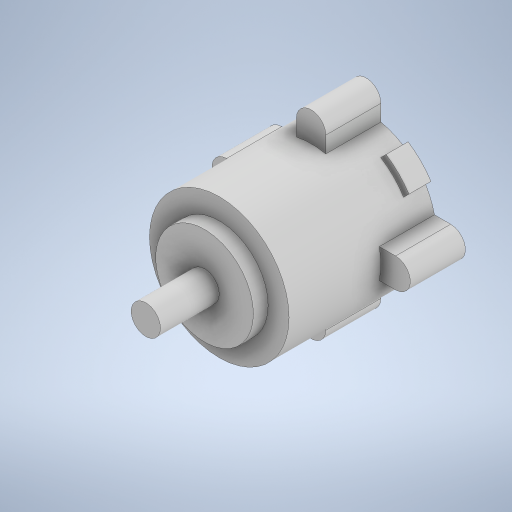
# Autodesk Inventor part: Solenoid Valve
Saved by Autodesk Inventor 2023 (Build 270158000, 158)
## iProperties
Created: 2024-03-20
Part Number: Solenoid Valve
Material: Generic
Document SubType Name: Modeling
Designer: Pobe Tran
Density: 1 g/cm^3
Appearance: Default
Author: Pobe Tran
Autodesk Inventor part; units mm, degrees
ref_plane "YZ Plane" through (0, 0, 0) normal (1, 0, 0) x (0, 1, 0)
ref_plane "XZ Plane" through (0, 0, 0) normal (0, 1, 0) x (-1, 0, 0)
ref_plane "XY Plane" through (0, 0, 0) normal (0, 0, 1) x (1, 0, 0)
sketch "Sketch1" plane through (0, 0, 0) normal (0, 0, 1) x (1, 0, 0)
  circle A0 centre (0, 0) radius 9.5
  arc A1 (2, 11.5) -> (-2, 11.5) centre (0, 11.5) ccw
  line L0 (-2, 11.5) -> (-2, 9.2871)
  line L1 (2, 11.5) -> (2, 9.2871)
  line L2 (11.5, -2) -> (9.2871, -2)
  arc A2 (11.5, -2) -> (11.5, 2) centre (11.5, 0) ccw
  line L3 (11.5, 2) -> (9.2871, 2)
  line L4 (-2, -11.5) -> (-2, -9.2871)
  arc A3 (-2, -11.5) -> (2, -11.5) centre (0, -11.5) ccw
  line L5 (2, -11.5) -> (2, -9.2871)
  line L6 (-11.5, 2) -> (-9.2871, 2)
  arc A4 (-11.5, 2) -> (-11.5, -2) centre (-11.5, 0) ccw
  line L7 (-11.5, -2) -> (-9.2871, -2)
  line L8 (0, 0) -> (6.7175, 6.7175) construction
  line L9 (0, 0) -> (9.5, 0) construction
  line L10 (5.7012, 8.8174) -> (4.9765, 8.0923)
  line L11 (8.8174, 5.7012) -> (8.0925, 4.9761)
  arc A5 (8.8174, 5.7012) -> (5.7012, 8.8174) centre (0, 0) ccw
  arc A6 (-10.3078, 2) -> (-10.3696, 1.6499) centre (0, 0) ccw
  arc A7 (-10.3696, -1.6499) -> (-10.3078, -2) centre (0, 0) ccw
  arc A8 (2, 10.3078) -> (1.6499, 10.3696) centre (0, 0) ccw
  arc A9 (-1.6499, 10.3696) -> (-2, 10.3078) centre (0, 0) ccw
  arc A10 (10.3078, -2) -> (10.5, 0) centre (0, 0) ccw
  arc A11 (10.3696, 1.6499) -> (10.3078, 2) centre (0, 0) ccw
  arc A12 (10.3078, -2) -> (10.3078, 2) centre (0, 0) ccw construction
  arc A13 (-2, -10.3078) -> (-1.6499, -10.3696) centre (0, 0) ccw
  arc A14 (1.6499, -10.3696) -> (2, -10.3078) centre (0, 0) ccw
  arc A15 (-2, -10.3078) -> (-1.6499, -10.3696) centre (0, 0) ccw construction
  arc A16 (1.6499, -10.3696) -> (2, -10.3078) centre (0, 0) ccw construction
  line L12 (-8.8174, -5.7012) -> (-8.0925, -4.9761)
  arc A17 (-8.8174, -5.7012) -> (-5.7012, -8.8174) centre (0, 0) ccw
  line L13 (-5.7012, -8.8174) -> (-4.9765, -8.0923)
  line L14 (7.4246, 7.4246) -> (0, 0) construction
  point P0 (-4.9765, -8.0923)
  dimension "d0" = 19
  dimension "d1" = 4
  dimension "d4" = 360
  dimension "d7" = 45
  dimension "d9" = 10.5
  dimension "d12" = 360
  constraints: 47 point on circle, 30 end point, 18 centre point, 10 point on line, 5 coincident, 3 tangent, 2 parallel, 1 equal length, 1 horizontal, 1 vertical, 1 vertical alignment, 52 other
  measures "d0" diameter of A0
  measures "d1" diameter of A1
  measures "d7" angle of L9 L8
  measures "d9" radius of A5
extrude "Extrusion1" add sketch "Sketch1" along normal blind 20 contours A0
extrude "Extrusion2" add sketch "Sketch1" along normal blind 7.5 contours A0 L3 A2 L2 | L5 A3 L4 A0 | A0 L0 A1 L1 | A0 L7 A4 L6
extrude "Extrusion3" add sketch "Sketch1" along normal blind 3 contours A0 L10 A5 L11 | L13 A17 L12 A0
sketch "Sketch2" plane through (0, 0, 20) normal (0, 0, 1) x (1, 0, 0)
  circle A0 centre (0, 0) radius 6.65
  dimension "d20" = 13.3
  constraints: 1 centre point, 1 coincident
  measures "d20" diameter of A0
extrude "Extrusion4" add sketch "Sketch2" along normal blind 2
sketch "Sketch3" plane through (0, 0, 22) normal (0, 0, 1) x (1, 0, 0)
  circle A0 centre (0, 0) radius 2
  dimension "d23" = 4
  constraints: 1 centre point, 1 coincident
  measures "d23" diameter of A0
extrude "Extrusion5" add sketch "Sketch3" along normal blind 8
body "Solid1"
